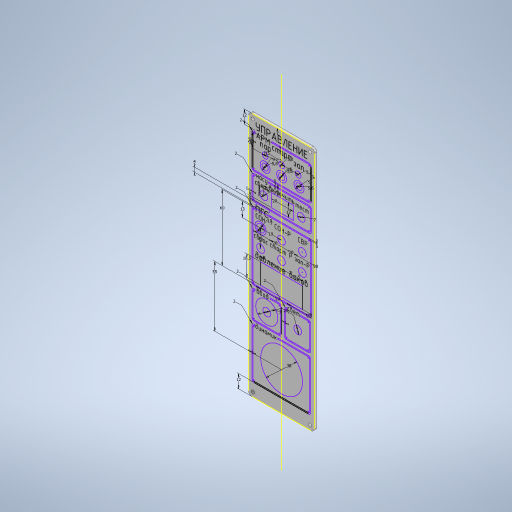
# Autodesk Inventor part: блок управления
Saved by Autodesk Inventor 2023.1 (Build 271208000, 208)
## iProperties
Created: 2023-02-23
Part Number: блок управления
Material: Типовые
Document SubType Name: Modeling
Designer: User
Density: 1 g/cm^3
Appearance: По умолчанию
Author: User
Autodesk Inventor part; units mm, degrees
ref_plane "YZ Plane" through (0, 0, 0) normal (1, 0, 0) x (0, 1, 0)
ref_plane "XZ Plane" through (0, 0, 0) normal (0, 1, 0) x (-1, 0, 0)
ref_plane "XY Plane" through (0, 0, 0) normal (0, 0, 1) x (1, 0, 0)
sketch "Эскиз1" plane through (0, 0, 0) normal (0, 0, 1) x (1, 0, 0)
  line L0 (-27, 111.5) -> (27, 111.5)
  line L1 (30, 108.5) -> (30, -108.5)
  line L2 (27, -111.5) -> (-27, -111.5)
  line L3 (-30, -108.5) -> (-30, 108.5)
  line L4 (0, -156.9698) -> (0, 156.9698) projected
  line L5 (-42.8698, 0) -> (42.8698, 0) projected
  arc A0 (-30, -108.5) -> (-27, -111.5) centre (-27, -108.5) ccw
  arc A1 (27, -111.5) -> (30, -108.5) centre (27, -108.5) ccw
  arc A2 (-27, 111.5) -> (-30, 108.5) centre (-27, 108.5) ccw
  arc A3 (30, 108.5) -> (27, 111.5) centre (27, 108.5) ccw
  circle A4 centre (-26, -107.5) radius 1.5
  circle A5 centre (26, -107.5) radius 1.5
  circle A6 centre (-26, 107.5) radius 1.5
  circle A7 centre (26, 107.5) radius 1.5
  point P0 (0, 0)
  dimension "d0" = 60
  dimension "d1" = 223
  dimension "d2" = 3
  dimension "d3" = 3
  dimension "d4" = 3
  dimension "d5" = 3
  dimension "d6" = 3
  dimension "d7" = 4
  dimension "d8" = 4
  dimension "d9" = 4
  dimension "d10" = 4
  dimension "d11" = 4
  dimension "d12" = 4
  dimension "d13" = 4
  dimension "d14" = 4
  constraints: 8 centre point, 8 end point, 8 point on circle, 8 tangent, 3 equal radius, 2 parallel, 1 horizontal, 1 perpendicular, 2 other
  measures "d0" distance between parallel lines of L1 L3
  measures "d1" distance between parallel lines of L2 L0
  measures "d2" radius of A0
  measures "d3" diameter of A4
  measures "d4" diameter of A5
  measures "d5" diameter of A6
  measures "d6" diameter of A7
  measures "d7" distance from line of L0 A6.centre
  measures "d8" distance from line of L3 A6.centre
  measures "d9" distance from line of L0 A7.centre
  measures "d10" distance from line of L1 A7.centre
  measures "d11" distance from line of L2 A5.centre
  measures "d12" distance from line of L1 A5.centre
  measures "d13" distance from line of L2 A4.centre
  measures "d14" distance from line of L3 A4.centre
extrude "Выдавливание1" add sketch "Эскиз1" along normal blind 2
sketch "Эскиз2" plane through (0, 0, 2) normal (0, 0, 1) x (1, 0, 0)
  line L0 (-23.9566, 106.5) -> (24.886, 106.5) construction
  line L1 (24.886, 106.5) -> (24.886, 99.5) construction
  line L2 (24.886, 99.5) -> (-23.9566, 99.5) construction
  line L3 (-23.9566, 99.5) -> (-23.9566, 106.5) construction
  line L4 (27, 111.5) -> (-27, 111.5) projected
  line L5 (27, 96.3309) -> (27, 69.0683)
  line L6 (25, 67.0683) -> (-25, 67.0683)
  line L7 (-27, 69.0683) -> (-27, 96.3309)
  line L8 (-30, 108.5) -> (-30, -108.5) projected
  line L9 (30, -108.5) -> (30, 108.5) projected
  circle A0 centre (-15, 84.3309) radius 2.6
  circle A1 centre (0, 84.3309) radius 2.6
  circle A2 centre (15, 84.3309) radius 2.6
  line L10 (-23.3416, 99.1446) -> (-10.9323, 99.1446) construction
  line L11 (-10.9323, 99.1446) -> (-10.9323, 96.0966) construction
  line L12 (-10.9323, 96.0966) -> (-23.3416, 96.0966) construction
  line L13 (-23.3416, 96.0966) -> (-23.3416, 99.1446) construction
  arc A3 (-25, 98.3309) -> (-27, 96.3309) centre (-25, 96.3309) ccw
  arc A4 (27, 96.3309) -> (25, 98.3309) centre (25, 96.3309) ccw
  arc A5 (25, 67.0683) -> (27, 69.0683) centre (25, 69.0683) ccw
  arc A6 (-27, 69.0683) -> (-25, 67.0683) centre (-25, 69.0683) ccw
  arc A7 (-25, 97.3309) -> (-26, 96.3309) centre (-25, 96.3309) ccw
  line L14 (-26, 96.3309) -> (-26, 69.0683)
  arc A8 (-26, 69.0683) -> (-25, 68.0683) centre (-25, 69.0683) ccw
  line L15 (-25, 68.0683) -> (25, 68.0683)
  arc A9 (25, 68.0683) -> (26, 69.0683) centre (25, 69.0683) ccw
  line L16 (26, 69.0683) -> (26, 96.3309)
  arc A10 (26, 96.3309) -> (25, 97.3309) centre (25, 96.3309) ccw
  line L17 (-23.9566, 98.3309) -> (-23.9566, 97.3309)
  line L18 (-8.9821, 98.3309) -> (-8.9821, 97.3309)
  line L19 (-25, 98.3309) -> (-23.9566, 98.3309)
  line L20 (-8.9821, 98.3309) -> (25, 98.3309)
  line L21 (25, 97.3309) -> (-8.9821, 97.3309)
  line L22 (-23.9566, 97.3309) -> (-25, 97.3309)
  line L23 (-8.9249, 95.3309) -> (1.4393, 95.3309) construction
  line L24 (1.4393, 95.3309) -> (1.4393, 92.1372) construction
  line L25 (1.4393, 92.1372) -> (-8.9249, 92.1372) construction
  line L26 (-8.9249, 92.1372) -> (-8.9249, 95.3309) construction
  line L27 (-19.7809, 92.8028) -> (-9.4167, 92.8028) construction
  line L28 (-9.4167, 92.8028) -> (-9.4167, 89.6091) construction
  line L29 (-9.4167, 89.6091) -> (-19.7809, 89.6091) construction
  line L30 (-19.7809, 89.6091) -> (-19.7809, 92.8028) construction
  line L31 (10.6082, 89.6091) -> (10.6082, 92.8028) construction
  line L32 (10.6082, 92.8028) -> (20.9724, 92.8028) construction
  line L33 (20.9724, 92.8028) -> (20.9724, 89.6091) construction
  line L34 (20.9724, 89.6091) -> (10.6082, 89.6091) construction
  circle A11 centre (-15, 75.2617) radius 2.8
  circle A12 centre (0, 75.2617) radius 2.8
  circle A13 centre (15.7903, 75.2617) radius 2.8
  circle A14 centre (-15, 75.2617) radius 4.5
  circle A15 centre (0, 75.2617) radius 4.5
  circle A16 centre (15.7903, 75.2617) radius 4.5
  line L35 (-9.1923, 58.0683) -> (10.8077, 58.0683)
  line L36 (10.8077, 58.0683) -> (10.8077, 46.0683)
  line L37 (10.8077, 46.0683) -> (-9.1923, 46.0683)
  line L38 (-9.1923, 46.0683) -> (-9.1923, 58.0683)
  line L39 (0, -156.1) -> (0, 156.1) projected
  circle A17 centre (-16.1923, 52.0683) radius 3.5
  circle A18 centre (17.8232, 52.0944) radius 3.5
  line L40 (26.9779, 63.0683) -> (26.9779, 45.0683)
  line L41 (24.9779, 43.0683) -> (-25.0088, 43.0683)
  line L42 (-27.0088, 45.0683) -> (-27.0088, 63.0683)
  arc A19 (-25.0088, 65.0683) -> (-27.0088, 63.0683) centre (-25.0088, 63.0683) ccw
  arc A20 (-27.0088, 45.0683) -> (-25.0088, 43.0683) centre (-25.0088, 45.0683) ccw
  arc A21 (24.9779, 43.0683) -> (26.9779, 45.0683) centre (24.9779, 45.0683) ccw
  arc A22 (26.9779, 63.0683) -> (24.9779, 65.0683) centre (24.9779, 63.0683) ccw
  line L43 (-24.3204, 57.95) -> (-24.3204, 61.1437) construction
  line L44 (-24.3204, 61.1437) -> (-13.9562, 61.1437) construction
  line L45 (-13.9562, 61.1437) -> (-13.9562, 57.95) construction
  line L46 (-13.9562, 57.95) -> (-24.3204, 57.95) construction
  arc A23 (-25.0088, 64.0683) -> (-26.0088, 63.0683) centre (-25.0088, 63.0683) ccw
  line L47 (-26.0088, 63.0683) -> (-26.0088, 45.0683)
  arc A24 (-26.0088, 45.0683) -> (-25.0088, 44.0683) centre (-25.0088, 45.0683) ccw
  line L48 (-25.0088, 44.0683) -> (24.9779, 44.0683)
  arc A25 (24.9779, 44.0683) -> (25.9779, 45.0683) centre (24.9779, 45.0683) ccw
  line L49 (25.9779, 45.0683) -> (25.9779, 63.0683)
  arc A26 (25.9779, 63.0683) -> (24.9779, 64.0683) centre (24.9779, 63.0683) ccw
  line L50 (12.5583, 57.4668) -> (12.5583, 60.6606) construction
  line L51 (12.5583, 60.6606) -> (22.9225, 60.6606) construction
  line L52 (22.9225, 60.6606) -> (22.9225, 57.4668) construction
  line L53 (22.9225, 57.4668) -> (12.5583, 57.4668) construction
  line L54 (-11.3578, 59.9059) -> (-11.3578, 63.0996) construction
  line L55 (-11.3578, 63.0996) -> (-0.9937, 63.0996) construction
  line L56 (-0.9937, 63.0996) -> (-0.9937, 59.9059) construction
  line L57 (-0.9937, 59.9059) -> (-11.3578, 59.9059) construction
  line L58 (27, 37.0683) -> (27, -20.9317)
  line L59 (25, -22.9317) -> (-25, -22.9317)
  line L60 (-27, -20.9317) -> (-27, 37.0683)
  arc A27 (-25, 39.0683) -> (-27, 37.0683) centre (-25, 37.0683) ccw
  arc A28 (27, 37.0683) -> (25, 39.0683) centre (25, 37.0683) ccw
  arc A29 (25, -22.9317) -> (27, -20.9317) centre (25, -20.9317) ccw
  arc A30 (-27, -20.9317) -> (-25, -22.9317) centre (-25, -20.9317) ccw
  line L61 (25, 38.0683) -> (-25, 38.0683)
  arc A31 (-25, 38.0683) -> (-26, 37.0683) centre (-25, 37.0683) ccw
  line L62 (-26, 37.0683) -> (-26, -20.9317)
  arc A32 (-26, -20.9317) -> (-25, -21.9317) centre (-25, -20.9317) ccw
  line L63 (-25, -21.9317) -> (25, -21.9317)
  arc A33 (25, -21.9317) -> (26, -20.9317) centre (25, -20.9317) ccw
  line L64 (26, -20.9317) -> (26, 37.0683)
  arc A34 (26, 37.0683) -> (25, 38.0683) centre (25, 37.0683) ccw
  line L65 (-23.9654, 65.0683) -> (-23.9654, 64.0683)
  line L66 (-12.2031, 65.0683) -> (-12.2031, 64.0683)
  line L67 (-25.0088, 65.0683) -> (-23.9654, 65.0683)
  line L68 (-12.2031, 65.0683) -> (24.9779, 65.0683)
  line L69 (24.9779, 64.0683) -> (-12.2031, 64.0683)
  line L70 (-23.9654, 64.0683) -> (-25.0088, 64.0683)
  line L71 (-23.2889, 65.7584) -> (-6.8733, 65.7584) construction
  line L72 (-6.8733, 65.7584) -> (-6.8733, 59.6787) construction
  line L73 (-6.8733, 59.6787) -> (-23.2889, 59.6787) construction
  line L74 (-23.2889, 59.6787) -> (-23.2889, 65.7584) construction
  line L75 (-23.6924, 31.7137) -> (-23.6924, 34.9075) construction
  line L76 (-23.6924, 34.9075) -> (-13.3282, 34.9075) construction
  line L77 (-13.3282, 34.9075) -> (-13.3282, 31.7137) construction
  line L78 (-13.3282, 31.7137) -> (-23.6924, 31.7137) construction
  circle A35 centre (-19.1383, 25.0683) radius 3.5
  circle A36 centre (-19.1383, 25.0683) radius 5
  circle A37 centre (-19.1383, 9.0683) radius 3.5
  circle A38 centre (-0.1383, 25.0683) radius 3.5
  circle A39 centre (-0.1383, 9.0683) radius 3.5
  circle A40 centre (18.8617, 25.0683) radius 3.5
  circle A41 centre (18.8617, 9.0683) radius 3.5
  line L79 (-6.528, 31.9598) -> (-6.528, 35.1535) construction
  line L80 (-6.528, 35.1535) -> (3.8362, 35.1535) construction
  line L81 (3.8362, 35.1535) -> (3.8362, 31.9598) construction
  line L82 (3.8362, 31.9598) -> (-6.528, 31.9598) construction
  line L83 (14.704, 32.139) -> (14.704, 35.3327) construction
  line L84 (14.704, 35.3327) -> (25.0682, 35.3327) construction
  line L85 (25.0682, 35.3327) -> (25.0682, 32.139) construction
  line L86 (25.0682, 32.139) -> (14.704, 32.139) construction
  line L87 (-25.321, 15.6293) -> (-25.321, 18.823) construction
  line L88 (-25.321, 18.823) -> (-5.321, 18.823) construction
  line L89 (-5.321, 18.823) -> (-5.321, 15.6293) construction
  line L90 (-5.321, 15.6293) -> (-25.321, 15.6293) construction
  line L91 (-10.7658, 15.5877) -> (-10.7658, 18.7814) construction
  line L92 (-10.7658, 18.7814) -> (9.2342, 18.7814) construction
  line L93 (9.2342, 18.7814) -> (9.2342, 15.5877) construction
  line L94 (9.2342, 15.5877) -> (-10.7658, 15.5877) construction
  line L95 (-4.17, 22.6618) -> (15.83, 22.6618) construction
  line L96 (11.6491, 15.7124) -> (11.6491, 18.9062) construction
  line L97 (11.6491, 18.9062) -> (31.6491, 18.9062) construction
  line L98 (31.6491, 18.9062) -> (31.6491, 15.7124) construction
  line L99 (31.6491, 15.7124) -> (11.6491, 15.7124) construction
  line L100 (-23.95, 39.0683) -> (-23.95, 38.0683)
  line L101 (-25, 39.0683) -> (-23.95, 39.0683)
  line L102 (-12.1876, 39.0683) -> (25, 39.0683)
  line L103 (-24.0093, 41.0623) -> (-11.7483, 41.0623) construction
  line L104 (-11.7483, 41.0623) -> (-11.7483, 35.884) construction
  line L105 (-11.7483, 35.884) -> (-24.0093, 35.884) construction
  line L106 (-24.0093, 35.884) -> (-24.0093, 41.0623) construction
  line L107 (-10.5, 39.0683) -> (-10.5, 38.0683)
  line L108 (-19.25, -1.4317) -> (19.25, -1.4317)
  line L109 (19.25, -1.4317) -> (19.25, -19.9317)
  line L110 (19.25, -19.9317) -> (-19.25, -19.9317)
  line L111 (-19.25, -19.9317) -> (-19.25, -1.4317)
  line L112 (-24.1108, 4.6891) -> (31.2098, 4.6891) construction
  line L113 (31.2098, 4.6891) -> (31.2098, -1.7888) construction
  line L114 (31.2098, -1.7888) -> (-24.1108, -1.7888) construction
  line L115 (-24.1108, -1.7888) -> (-24.1108, 4.6891) construction
  line L116 (0, -27.439) -> (0, -49.021)
  line L117 (-2, -51.021) -> (-25, -51.021)
  line L118 (-27, -49.021) -> (-27, -27.439)
  circle A42 centre (-13.5, -38.23) radius 10
  arc A43 (-25, -25.439) -> (-27, -27.439) centre (-25, -27.439) ccw
  arc A44 (0, -27.439) -> (-2, -25.439) centre (-2, -27.439) ccw
  arc A45 (-2, -51.021) -> (0, -49.021) centre (-2, -49.021) ccw
  arc A46 (-27, -49.021) -> (-25, -51.021) centre (-25, -49.021) ccw
  arc A47 (-25, -26.439) -> (-26, -27.439) centre (-25, -27.439) ccw
  line L119 (-26, -27.439) -> (-26, -49.021)
  arc A48 (-26, -49.021) -> (-25, -50.021) centre (-25, -49.021) ccw
  line L120 (-25, -50.021) -> (-2, -50.021)
  arc A49 (-2, -50.021) -> (-1, -49.021) centre (-2, -49.021) ccw
  line L121 (-1, -49.021) -> (-1, -27.439)
  arc A50 (-1, -27.439) -> (-2, -26.439) centre (-2, -27.439) ccw
  line L122 (-24.1108, -26.439) -> (-24.1108, -25.439)
  line L123 (-22.836, -27.0695) -> (-22.836, -23.8757) construction
  line L124 (-22.836, -23.8757) -> (-2.836, -23.8757) construction
  line L125 (-2.836, -23.8757) -> (-2.836, -27.0695) construction
  line L126 (-2.836, -27.0695) -> (-22.836, -27.0695) construction
  line L127 (-10.5, -26.439) -> (-10.5, -25.439)
  line L128 (-25, -25.439) -> (-24.1108, -25.439)
  line L129 (-10.5, -25.439) -> (-2, -25.439)
  line L130 (-2, -26.439) -> (-10.5, -26.439)
  line L131 (-24.1108, -26.439) -> (-25, -26.439)
  circle A51 centre (-13.5, -38.23) radius 3.5
  circle A52 centre (0, -76.9317) radius 19
  line L132 (26.4142, -55.5075) -> (26.4142, -97.5)
  line L133 (24.4142, -99.5) -> (-25, -99.5)
  line L134 (-27, -97.5) -> (-27, -55.5075)
  line L135 (-27, -111.5) -> (27, -111.5) projected
  arc A53 (-25, -53.5075) -> (-27, -55.5075) centre (-25, -55.5075) ccw
  arc A54 (26.4142, -55.5075) -> (24.4142, -53.5075) centre (24.4142, -55.5075) ccw
  arc A55 (-27, -97.5) -> (-25, -99.5) centre (-25, -97.5) ccw
  arc A56 (24.4142, -99.5) -> (26.4142, -97.5) centre (24.4142, -97.5) ccw
  line L136 (-26, -55.5075) -> (-26, -97.5)
  arc A57 (-26, -97.5) -> (-25, -98.5) centre (-25, -97.5) ccw
  line L137 (-25, -98.5) -> (24.4142, -98.5)
  arc A58 (24.4142, -98.5) -> (25.4142, -97.5) centre (24.4142, -97.5) ccw
  line L138 (25.4142, -97.5) -> (25.4142, -55.5075)
  arc A59 (25.4142, -55.5075) -> (24.4142, -54.5075) centre (24.4142, -55.5075) ccw
  arc A60 (-25, -54.5075) -> (-26, -55.5075) centre (-25, -55.5075) ccw
  line L139 (-24.475, -54.5075) -> (-24.475, -53.5075)
  line L140 (-23.9774, -52.0239) -> (-4.0406, -52.0239) construction
  line L141 (-4.0406, -52.0239) -> (-4.0406, -56.0172) construction
  line L142 (-4.0406, -56.0172) -> (-23.9774, -56.0172) construction
  line L143 (-23.9774, -56.0172) -> (-23.9774, -52.0239) construction
  line L144 (-3.5, -54.5075) -> (-3.5, -53.5075)
  line L145 (-25, -53.5075) -> (-24.475, -53.5075)
  line L146 (-3.5, -53.5075) -> (24.4142, -53.5075)
  line L147 (24.4142, -54.5075) -> (-3.5, -54.5075)
  line L148 (-24.475, -54.5075) -> (-25, -54.5075)
  line L149 (26.4142, -27.439) -> (26.4142, -49.021)
  line L150 (24.4142, -51.021) -> (4.8, -51.021)
  line L151 (2.8, -49.021) -> (2.8, -27.439)
  arc A61 (4.8, -25.439) -> (2.8, -27.439) centre (4.8, -27.439) ccw
  arc A62 (26.4142, -27.439) -> (24.4142, -25.439) centre (24.4142, -27.439) ccw
  arc A63 (2.8, -49.021) -> (4.8, -51.021) centre (4.8, -49.021) ccw
  arc A64 (24.4142, -51.021) -> (26.4142, -49.021) centre (24.4142, -49.021) ccw
  line L152 (3.8, -27.439) -> (3.8, -49.021)
  arc A65 (3.8, -49.021) -> (4.8, -50.021) centre (4.8, -49.021) ccw
  line L153 (4.8, -50.021) -> (24.4142, -50.021)
  arc A66 (24.4142, -50.021) -> (25.4142, -49.021) centre (24.4142, -49.021) ccw
  line L154 (25.4142, -49.021) -> (25.4142, -27.439)
  arc A67 (25.4142, -27.439) -> (24.4142, -26.439) centre (24.4142, -27.439) ccw
  arc A68 (4.8, -26.439) -> (3.8, -27.439) centre (4.8, -27.439) ccw
  line L155 (4.8, -25.439) -> (4.8, -26.439)
  line L156 (5.2245, -26.5009) -> (5.2245, -23.3071) construction
  line L157 (5.2245, -23.3071) -> (25.2245, -23.3071) construction
  line L158 (25.2245, -23.3071) -> (25.2245, -26.5009) construction
  line L159 (25.2245, -26.5009) -> (5.2245, -26.5009) construction
  line L160 (17.2098, -26.439) -> (17.2098, -25.439)
  line L161 (4.8, -25.439) -> (4.9172, -25.439)
  line L162 (17.2098, -25.439) -> (24.4142, -25.439)
  line L163 (24.4142, -26.439) -> (17.2098, -26.439)
  line L164 (4.9172, -26.439) -> (4.8, -26.439)
  circle A69 centre (14.6071, -38.23) radius 3.5
  point P0 (0, 0)
  point P1 (-22.95, 41.759)
  point P2 (-11.1876, 41.759)
  point P3 (0, -51.021)
  dimension "d17" = 5
  dimension "d18" = 3
  dimension "d19" = 3
  dimension "d20" = 12
  dimension "d21" = 5.2
  dimension "d22" = 5.2
  dimension "d23" = 5.2
  dimension "d25" = 2
  dimension "d28" = 15
  dimension "d29" = 15
  dimension "d30" = 13
  dimension "d31" = 2
  dimension "d32" = 5.6
  dimension "d33" = 5.6
  dimension "d34" = 5.6
  dimension "d35" = 9
  dimension "d36" = 9
  dimension "d37" = 9
  dimension "d38" = 12
  dimension "d39" = 20
  dimension "d40" = 7
  dimension "d41" = 7
  dimension "d42" = 7
  dimension "d44" = 9
  dimension "d45" = 6
  dimension "d46" = 2
  dimension "d48" = 2
  dimension "d50" = 2
  dimension "d51" = 2
  dimension "d53" = 1
  dimension "d54" = 7
  dimension "d55" = 10
  dimension "d56" = 13
  dimension "d59" = 16
  dimension "d62" = 19
  dimension "d65" = 60
  dimension "d66" = 20
  dimension "d67" = 20
  dimension "d68" = 20
  dimension "d69" = 4
  dimension "d70" = 1
  dimension "d71" = 1
  dimension "d73" = 38.5
  dimension "d74" = 18.5
  dimension "d75" = 2
  dimension "d76" = 20
  dimension "d77" = 2
  dimension "d79" = 20
  dimension "d80" = 7
  dimension "d81" = 38
  dimension "d82" = 55
  dimension "d83" = 12
  dimension "d84" = 2
  dimension "d85" = 1
  dimension "d86" = 2
  dimension "d87" = 1
  dimension "d88" = 20
  dimension "d89" = 7
  constraints: 158 end point, 96 point on circle, 70 centre point, 60 tangent, 45 perpendicular, 39 parallel, 18 equal radius, 15 horizontal, 7 point on line, 5 coincident, 3 horizontal alignment, 1 vertical, 1 vertical alignment, 85 other
  measures "d17" distance between parallel lines of L4 L0
  measures "d18" distance between parallel lines of L7 L8
  measures "d19" distance between parallel lines of L9 L5
  measures "d20" distance between parallel lines of L4 L2
  measures "d21" diameter of A0
  measures "d22" diameter of A1
  measures "d23" diameter of A2
  measures "d25" radius of A3
  measures "d28" distance of A0.centre A1.centre
  measures "d29" distance of A1.centre A2.centre
  measures "d30" distance from line of L21 A0.centre
  measures "d31" distance between parallel lines of L21 L23
  measures "d32" diameter of A11
  measures "d33" diameter of A12
  measures "d34" diameter of A13
  measures "d35" diameter of A14
  measures "d36" diameter of A15
  measures "d37" diameter of A16
  measures "d38" distance between parallel lines of L35 L37
  measures "d39" distance between parallel lines of L38 L36
  measures "d40" diameter of A17
  measures "d41" diameter of A18
  measures "d42" distance from line of L38 A17.centre
  measures "d44" distance between parallel lines of L35 L6
  measures "d45" distance from line of A17.centre L35
  measures "d46" radius of A19
  measures "d48" radius of A27
  measures "d50" distance between parallel lines of L6 L68
  measures "d51" distance between parallel lines of L37 L48
  measures "d53" distance between parallel lines of L7 L14
  measures "d54" diameter of A35
  measures "d55" diameter of A36
  measures "d56" distance from line of L61 A35.centre
  measures "d59" distance of A35.centre A37.centre
  measures "d62" distance of A35.centre A38.centre
  measures "d65" distance between parallel lines of L61 L63
  measures "d66" distance between parallel lines of L89 L87
  measures "d67" distance between parallel lines of L93 L91
  measures "d68" distance between parallel lines of L98 L96
  measures "d69" distance between parallel lines of L102 L41
  measures "d70" distance between parallel lines of L42 L47
  measures "d71" distance between parallel lines of L61 L102
  measures "d73" distance between parallel lines of L109 L111
  measures "d74" distance between parallel lines of L108 L110
  measures "d75" distance between parallel lines of L63 L110
  measures "d76" diameter of A42
  measures "d77" radius of A43
  measures "d79" distance between parallel lines of L125 L123
  measures "d80" diameter of A51
  measures "d81" diameter of A52
  measures "d82" distance from line of L63 A52.centre
  measures "d83" distance between parallel lines of L133 L135
  measures "d84" radius of A53
  measures "d85" distance between parallel lines of L134 L136
  measures "d86" radius of A61
  measures "d87" distance between parallel lines of L151 L152
  measures "d88" distance between parallel lines of L158 L156
  measures "d89" diameter of A69
